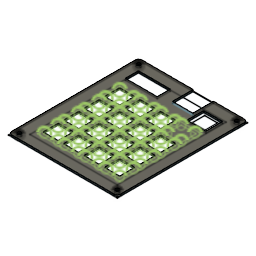
final (Autodesk Fusion 360 archive; units mm, degrees)
design "top"
part number: 2025-12-10-00-46-04-240
Autodesk Fusion 360 part; units mm, degrees
sketch "plate-2025-12-08T02_56_49.771Z" plane through (0, 0, 0) normal (0, 0, 1) x (1, 0, 0)
  line L0 (3.025, -2.525) -> (16.025, -2.525)
  line L1 (3.025, -16.525) -> (16.025, -16.525)
  line L2 (2.525, -3.025) -> (2.525, -16.025)
  line L3 (16.525, -3.025) -> (16.525, -16.025)
  arc A0 (3.025, -2.525) -> (2.525, -3.025) centre (3.025, -3.025) ccw
  arc A1 (16.525, -3.025) -> (16.025, -2.525) centre (16.025, -3.025) ccw
  arc A2 (2.525, -16.025) -> (3.025, -16.525) centre (3.025, -16.025) ccw
  arc A3 (16.025, -16.525) -> (16.525, -16.025) centre (16.025, -16.025) ccw
  line L4 (22.075, -2.525) -> (35.075, -2.525)
  line L5 (22.075, -16.525) -> (35.075, -16.525)
  line L6 (21.575, -3.025) -> (21.575, -16.025)
  line L7 (35.575, -3.025) -> (35.575, -16.025)
  arc A4 (22.075, -2.525) -> (21.575, -3.025) centre (22.075, -3.025) ccw
  arc A5 (35.575, -3.025) -> (35.075, -2.525) centre (35.075, -3.025) ccw
  arc A6 (21.575, -16.025) -> (22.075, -16.525) centre (22.075, -16.025) ccw
  arc A7 (35.075, -16.525) -> (35.575, -16.025) centre (35.075, -16.025) ccw
  line L8 (41.125, -2.525) -> (54.125, -2.525)
  line L9 (41.125, -16.525) -> (54.125, -16.525)
  line L10 (40.625, -3.025) -> (40.625, -16.025)
  line L11 (54.625, -3.025) -> (54.625, -16.025)
  arc A8 (41.125, -2.525) -> (40.625, -3.025) centre (41.125, -3.025) ccw
  arc A9 (54.625, -3.025) -> (54.125, -2.525) centre (54.125, -3.025) ccw
  arc A10 (40.625, -16.025) -> (41.125, -16.525) centre (41.125, -16.025) ccw
  arc A11 (54.125, -16.525) -> (54.625, -16.025) centre (54.125, -16.025) ccw
  line L12 (60.175, -2.525) -> (73.175, -2.525)
  line L13 (60.175, -16.525) -> (73.175, -16.525)
  line L14 (59.675, -3.025) -> (59.675, -16.025)
  line L15 (73.675, -3.025) -> (73.675, -16.025)
  arc A12 (60.175, -2.525) -> (59.675, -3.025) centre (60.175, -3.025) ccw
  arc A13 (73.675, -3.025) -> (73.175, -2.525) centre (73.175, -3.025) ccw
  arc A14 (59.675, -16.025) -> (60.175, -16.525) centre (60.175, -16.025) ccw
  arc A15 (73.175, -16.525) -> (73.675, -16.025) centre (73.175, -16.025) ccw
  line L16 (3.025, -21.575) -> (16.025, -21.575)
  line L17 (3.025, -35.575) -> (16.025, -35.575)
  line L18 (2.525, -22.075) -> (2.525, -35.075)
  line L19 (16.525, -22.075) -> (16.525, -35.075)
  arc A16 (3.025, -21.575) -> (2.525, -22.075) centre (3.025, -22.075) ccw
  arc A17 (16.525, -22.075) -> (16.025, -21.575) centre (16.025, -22.075) ccw
  arc A18 (2.525, -35.075) -> (3.025, -35.575) centre (3.025, -35.075) ccw
  arc A19 (16.025, -35.575) -> (16.525, -35.075) centre (16.025, -35.075) ccw
  line L20 (22.075, -21.575) -> (35.075, -21.575)
  line L21 (22.075, -35.575) -> (35.075, -35.575)
  line L22 (21.575, -22.075) -> (21.575, -35.075)
  line L23 (35.575, -22.075) -> (35.575, -35.075)
  arc A20 (22.075, -21.575) -> (21.575, -22.075) centre (22.075, -22.075) ccw
  arc A21 (35.575, -22.075) -> (35.075, -21.575) centre (35.075, -22.075) ccw
  arc A22 (21.575, -35.075) -> (22.075, -35.575) centre (22.075, -35.075) ccw
  arc A23 (35.075, -35.575) -> (35.575, -35.075) centre (35.075, -35.075) ccw
  line L24 (41.125, -21.575) -> (54.125, -21.575)
  line L25 (41.125, -35.575) -> (54.125, -35.575)
  line L26 (40.625, -22.075) -> (40.625, -35.075)
  line L27 (54.625, -22.075) -> (54.625, -35.075)
  arc A24 (41.125, -21.575) -> (40.625, -22.075) centre (41.125, -22.075) ccw
  arc A25 (54.625, -22.075) -> (54.125, -21.575) centre (54.125, -22.075) ccw
  arc A26 (40.625, -35.075) -> (41.125, -35.575) centre (41.125, -35.075) ccw
  arc A27 (54.125, -35.575) -> (54.625, -35.075) centre (54.125, -35.075) ccw
  line L28 (60.175, -21.575) -> (73.175, -21.575)
  line L29 (60.175, -35.575) -> (73.175, -35.575)
  line L30 (59.675, -22.075) -> (59.675, -35.075)
  line L31 (73.675, -22.075) -> (73.675, -35.075)
  arc A28 (60.175, -21.575) -> (59.675, -22.075) centre (60.175, -22.075) ccw
  arc A29 (73.675, -22.075) -> (73.175, -21.575) centre (73.175, -22.075) ccw
  arc A30 (59.675, -35.075) -> (60.175, -35.575) centre (60.175, -35.075) ccw
  arc A31 (73.175, -35.575) -> (73.675, -35.075) centre (73.175, -35.075) ccw
  line L32 (3.025, -40.625) -> (16.025, -40.625)
  line L33 (3.025, -54.625) -> (16.025, -54.625)
  line L34 (2.525, -41.125) -> (2.525, -54.125)
  line L35 (16.525, -41.125) -> (16.525, -54.125)
  arc A32 (3.025, -40.625) -> (2.525, -41.125) centre (3.025, -41.125) ccw
  arc A33 (16.525, -41.125) -> (16.025, -40.625) centre (16.025, -41.125) ccw
  arc A34 (2.525, -54.125) -> (3.025, -54.625) centre (3.025, -54.125) ccw
  arc A35 (16.025, -54.625) -> (16.525, -54.125) centre (16.025, -54.125) ccw
  line L36 (22.075, -40.625) -> (35.075, -40.625)
  line L37 (22.075, -54.625) -> (35.075, -54.625)
  line L38 (21.575, -41.125) -> (21.575, -54.125)
  line L39 (35.575, -41.125) -> (35.575, -54.125)
  arc A36 (22.075, -40.625) -> (21.575, -41.125) centre (22.075, -41.125) ccw
  arc A37 (35.575, -41.125) -> (35.075, -40.625) centre (35.075, -41.125) ccw
  arc A38 (21.575, -54.125) -> (22.075, -54.625) centre (22.075, -54.125) ccw
  arc A39 (35.075, -54.625) -> (35.575, -54.125) centre (35.075, -54.125) ccw
  line L40 (41.125, -40.625) -> (54.125, -40.625)
  line L41 (41.125, -54.625) -> (54.125, -54.625)
  line L42 (40.625, -41.125) -> (40.625, -54.125)
  line L43 (54.625, -41.125) -> (54.625, -54.125)
  arc A40 (41.125, -40.625) -> (40.625, -41.125) centre (41.125, -41.125) ccw
  arc A41 (54.625, -41.125) -> (54.125, -40.625) centre (54.125, -41.125) ccw
  arc A42 (40.625, -54.125) -> (41.125, -54.625) centre (41.125, -54.125) ccw
  arc A43 (54.125, -54.625) -> (54.625, -54.125) centre (54.125, -54.125) ccw
  line L44 (60.175, -40.625) -> (73.175, -40.625)
  line L45 (60.175, -54.625) -> (73.175, -54.625)
  line L46 (59.675, -41.125) -> (59.675, -54.125)
  line L47 (73.675, -41.125) -> (73.675, -54.125)
  arc A44 (60.175, -40.625) -> (59.675, -41.125) centre (60.175, -41.125) ccw
  arc A45 (73.675, -41.125) -> (73.175, -40.625) centre (73.175, -41.125) ccw
  arc A46 (59.675, -54.125) -> (60.175, -54.625) centre (60.175, -54.125) ccw
  arc A47 (73.175, -54.625) -> (73.675, -54.125) centre (73.175, -54.125) ccw
  line L48 (3.025, -59.675) -> (16.025, -59.675)
  line L49 (3.025, -73.675) -> (16.025, -73.675)
  line L50 (2.525, -60.175) -> (2.525, -73.175)
  line L51 (16.525, -60.175) -> (16.525, -73.175)
  arc A48 (3.025, -59.675) -> (2.525, -60.175) centre (3.025, -60.175) ccw
  arc A49 (16.525, -60.175) -> (16.025, -59.675) centre (16.025, -60.175) ccw
  arc A50 (2.525, -73.175) -> (3.025, -73.675) centre (3.025, -73.175) ccw
  arc A51 (16.025, -73.675) -> (16.525, -73.175) centre (16.025, -73.175) ccw
  line L52 (22.075, -59.675) -> (35.075, -59.675)
  line L53 (22.075, -73.675) -> (35.075, -73.675)
  line L54 (21.575, -60.175) -> (21.575, -73.175)
  line L55 (35.575, -60.175) -> (35.575, -73.175)
  arc A52 (22.075, -59.675) -> (21.575, -60.175) centre (22.075, -60.175) ccw
  arc A53 (35.575, -60.175) -> (35.075, -59.675) centre (35.075, -60.175) ccw
  arc A54 (21.575, -73.175) -> (22.075, -73.675) centre (22.075, -73.175) ccw
  arc A55 (35.075, -73.675) -> (35.575, -73.175) centre (35.075, -73.175) ccw
  line L56 (41.125, -59.675) -> (54.125, -59.675)
  line L57 (41.125, -73.675) -> (54.125, -73.675)
  line L58 (40.625, -60.175) -> (40.625, -73.175)
  line L59 (54.625, -60.175) -> (54.625, -73.175)
  arc A56 (41.125, -59.675) -> (40.625, -60.175) centre (41.125, -60.175) ccw
  arc A57 (54.625, -60.175) -> (54.125, -59.675) centre (54.125, -60.175) ccw
  arc A58 (40.625, -73.175) -> (41.125, -73.675) centre (41.125, -73.175) ccw
  arc A59 (54.125, -73.675) -> (54.625, -73.175) centre (54.125, -73.175) ccw
  line L60 (60.175, -59.675) -> (73.175, -59.675)
  line L61 (60.175, -73.675) -> (73.175, -73.675)
  line L62 (59.675, -60.175) -> (59.675, -73.175)
  line L63 (73.675, -60.175) -> (73.675, -73.175)
  arc A60 (60.175, -59.675) -> (59.675, -60.175) centre (60.175, -60.175) ccw
  arc A61 (73.675, -60.175) -> (73.175, -59.675) centre (73.175, -60.175) ccw
  arc A62 (59.675, -73.175) -> (60.175, -73.675) centre (60.175, -73.175) ccw
  arc A63 (73.175, -73.675) -> (73.675, -73.175) centre (73.175, -73.175) ccw
  line L64 (0, -76.2) -> (76.2, -76.2)
  line L65 (0, 0) -> (76.2, 0)
  line L66 (0, -76.2) -> (0, 0)
  line L67 (76.2, -76.2) -> (76.2, 0)
  line L68 (-2.995, 20.635) -> (78.195, 20.635)
  line L69 (78.195, 20.635) -> (78.195, -80.365)
  line L70 (78.195, -80.365) -> (-2.995, -80.365)
  line L71 (-2.995, -80.365) -> (-2.995, 20.635)
  line L72 (62.965, 16.055) -> (74.965, 16.055)
  line L73 (74.965, 16.055) -> (74.965, 4.455)
  line L74 (74.965, 4.455) -> (62.965, 4.455)
  line L75 (62.965, 4.455) -> (62.965, 16.055)
  line L76 (60.065, 18.055) -> (77.565, 18.055)
  line L77 (77.565, 18.055) -> (77.565, 2.655)
  line L78 (77.565, 2.655) -> (60.065, 2.655)
  line L79 (60.065, 2.655) -> (60.065, 18.055)
  line L80 (-2.28, 19.7) -> (27.22, 19.7)
  line L81 (27.22, 19.7) -> (27.22, 7.7)
  line L82 (27.22, 7.7) -> (-2.28, 7.7)
  line L83 (-2.28, 7.7) -> (-2.28, 19.7)
  line L84 (-12.495, 30.135) -> (88.695, 30.135)
  line L85 (88.695, 30.135) -> (88.695, -90.865)
  line L86 (88.695, -90.865) -> (-12.495, -90.865)
  line L87 (-12.495, -90.865) -> (-12.495, 30.135)
  circle A64 centre (-7.495, 25.135) radius 1.7
  circle A65 centre (-7.495, -85.865) radius 1.7
  circle A66 centre (83.695, -85.865) radius 1.7
  circle A67 centre (83.695, 25.135) radius 1.7
  line L88 (38.235, 30.135) -> (57.064, 30.135)
  line L89 (57.064, 30.135) -> (57.064, 11)
  line L90 (57.064, 11) -> (38.235, 11)
  line L91 (38.235, 11) -> (38.235, 30.135)
  dimension "d3" = 101
  dimension "d4" = 81.19
  dimension "d6" = 1.995
  dimension "d7" = 4.165
  dimension "d11" = 12
  dimension "d12" = 11.6
  dimension "d16" = 15.4
  dimension "d17" = 17.5
  dimension "d18" = 2.9
  dimension "d19" = 1.8
  dimension "d22" = 29.5
  dimension "d23" = 12
  dimension "d25" = 0.935
  dimension "d29" = 0.715
  dimension "d33" = 9.5
  dimension "d34" = 3.4
  dimension "d35" = 5
  dimension "d36" = 5
  dimension "d37" = 3.4
  dimension "d38" = 5
  dimension "d39" = 5
  dimension "d40" = 3.4
  dimension "d41" = 5
  dimension "d42" = 5
  dimension "d43" = 3.4
  dimension "d44" = 5
  dimension "d45" = 5
  dimension "d46" = 41.23
  dimension "d48" = 21.131
  dimension "d49" = 18.829
  dimension "d53" = 2.58
  dimension "d55" = 0.63
  dimension "d65" = 121
  dimension "d66" = 9.5
  dimension "d67" = 10.5
  constraint horizontal L68
  constraint vertical L69
  constraint horizontal L70
  constraint vertical L71
  constraint horizontal L72
  constraint vertical L73
  constraint horizontal L74
  constraint vertical L75
  constraint horizontal L76
  constraint vertical L77
  constraint horizontal L78
  constraint vertical L79
  constraint horizontal L80
  constraint vertical L81
  constraint horizontal L82
  constraint vertical L83
  constraint horizontal L84
  constraint vertical L85
  constraint horizontal L86
  constraint vertical L87
  constraint horizontal L88
  constraint vertical L89
  constraint horizontal L90
  constraint vertical L91
  constraint coincident L84 L88.start
  measures "d3" distance of L68.end L69.end
  measures "d4" distance of L69.end L70.end
  measures "d6" distance of L67 L69
  measures "d7" distance of L64 L70
  measures "d11" distance of L72.start L72.end
  measures "d12" distance of L72.start L74.end
  measures "d16" distance of L76.start L78.end
  measures "d17" distance of L77.end L78.end
  measures "d18" distance of L75 L79
  measures "d19" distance of L74 L78
  measures "d22" distance of L81.end L82.end
  measures "d23" distance of L80.end L81.end
  measures "d25" distance of L68 L80
  measures "d29" distance of L71 L83
  measures "d33" distance of L68 L84
  measures "d34" diameter of A64
  measures "d35" distance of L84 A64.centre
  measures "d36" distance of L87 A64.centre
  measures "d37" diameter of A65
  measures "d38" distance of L86 A65.centre
  measures "d39" distance of L87 A65.centre
  measures "d40" diameter of A66
  measures "d41" distance of L86 A66.centre
  measures "d42" distance of L85 A66.centre
  measures "d43" diameter of A67
  measures "d44" distance of L84 A67.centre
  measures "d45" distance of L85 A67.centre
  measures "d46" distance of L71 L90.end
  measures "d48" distance of L69 L89.end
  measures "d49" distance of L89.end L90.end
  measures "d53" vertical distance of L68.end L76.end
  measures "d55" distance of L69 L77
  measures "d65" distance of L84.end L85.end
  measures "d66" distance of L71 L87
  measures "d67" distance of L69 L85
extrude "Extrude1" add sketch "plate-2025-12-08T02_56_49.771Z" along normal blind 1.5 contours L68 L69 L70 L71 L89 L90 L91
extrude "Extrude2" add sketch "plate-2025-12-08T02_56_49.771Z" along normal blind 1.5 contours L68 L69 L70 L71 L84 L85 L86 L87 L89 L91
extrude "Extrude3" add sketch "plate-2025-12-08T02_56_49.771Z" along normal blind 1.5 contours L64 L65 L66 L67
fillet "Fillet1" radius 3 4 edges at (88.695, -90.865, 0.75) (88.695, 30.135, 0.75) (-12.495, 30.135, 0.75) (-12.495, -90.865, 0.75)
sketch "Sketch2" plane through (0, 0, 1.5) normal (0, 0, 1) x (1, 0, 0)
sketch "Sketch3" plane through (0, 0, 1.5) normal (0, 0, 1) x (-1, 0, 0)
  arc A0 (12.495, 87.865) -> (9.495, 90.865) centre (9.495, 87.865) ccw
  line L0 (9.495, 90.865) -> (-85.695, 90.865)
  arc A1 (-85.695, 90.865) -> (-88.695, 87.865) centre (-85.695, 87.865) ccw
  line L1 (-88.695, 87.865) -> (-88.695, -27.135)
  arc A2 (-88.695, -27.135) -> (-85.695, -30.135) centre (-85.695, -27.135) ccw
  line L2 (-85.695, -30.135) -> (-57.064, -30.135)
  line L3 (-57.064, -30.135) -> (-57.064, -11)
  line L4 (-57.064, -11) -> (-38.235, -11)
  line L5 (-38.235, -11) -> (-38.235, -30.135)
  line L6 (-38.235, -30.135) -> (9.495, -30.135)
  arc A3 (9.495, -30.135) -> (12.495, -27.135) centre (9.495, -27.135) ccw
  line L7 (12.495, -27.135) -> (12.495, 87.865)
  arc A4 (-41.125, 2.525) -> (-40.625, 3.025) centre (-41.125, 3.025) ccw
  line L8 (-41.125, 2.525) -> (-54.125, 2.525)
  arc A5 (-54.625, 3.025) -> (-54.125, 2.525) centre (-54.125, 3.025) ccw
  line L9 (-54.625, 3.025) -> (-54.625, 16.025)
  arc A6 (-54.125, 16.525) -> (-54.625, 16.025) centre (-54.125, 16.025) ccw
  line L10 (-54.125, 16.525) -> (-41.125, 16.525)
  arc A7 (-40.625, 16.025) -> (-41.125, 16.525) centre (-41.125, 16.025) ccw
  line L11 (-40.625, 16.025) -> (-40.625, 3.025)
  arc A8 (-3.025, 59.675) -> (-2.525, 60.175) centre (-3.025, 60.175) ccw
  line L12 (-3.025, 59.675) -> (-16.025, 59.675)
  arc A9 (-16.525, 60.175) -> (-16.025, 59.675) centre (-16.025, 60.175) ccw
  line L13 (-16.525, 60.175) -> (-16.525, 73.175)
  arc A10 (-16.025, 73.675) -> (-16.525, 73.175) centre (-16.025, 73.175) ccw
  line L14 (-16.025, 73.675) -> (-3.025, 73.675)
  arc A11 (-2.525, 73.175) -> (-3.025, 73.675) centre (-3.025, 73.175) ccw
  line L15 (-2.525, 73.175) -> (-2.525, 60.175)
  arc A12 (-60.175, 2.525) -> (-59.675, 3.025) centre (-60.175, 3.025) ccw
  line L16 (-60.175, 2.525) -> (-73.175, 2.525)
  arc A13 (-73.675, 3.025) -> (-73.175, 2.525) centre (-73.175, 3.025) ccw
  line L17 (-73.675, 3.025) -> (-73.675, 16.025)
  arc A14 (-73.175, 16.525) -> (-73.675, 16.025) centre (-73.175, 16.025) ccw
  line L18 (-73.175, 16.525) -> (-60.175, 16.525)
  arc A15 (-59.675, 16.025) -> (-60.175, 16.525) centre (-60.175, 16.025) ccw
  line L19 (-59.675, 16.025) -> (-59.675, 3.025)
  arc A16 (-22.075, 21.575) -> (-21.575, 22.075) centre (-22.075, 22.075) ccw
  line L20 (-22.075, 21.575) -> (-35.075, 21.575)
  arc A17 (-35.575, 22.075) -> (-35.075, 21.575) centre (-35.075, 22.075) ccw
  line L21 (-35.575, 22.075) -> (-35.575, 35.075)
  arc A18 (-35.075, 35.575) -> (-35.575, 35.075) centre (-35.075, 35.075) ccw
  line L22 (-35.075, 35.575) -> (-22.075, 35.575)
  arc A19 (-21.575, 35.075) -> (-22.075, 35.575) centre (-22.075, 35.075) ccw
  line L23 (-21.575, 35.075) -> (-21.575, 22.075)
  arc A20 (-41.125, 40.625) -> (-40.625, 41.125) centre (-41.125, 41.125) ccw
  line L24 (-41.125, 40.625) -> (-54.125, 40.625)
  arc A21 (-54.625, 41.125) -> (-54.125, 40.625) centre (-54.125, 41.125) ccw
  line L25 (-54.625, 41.125) -> (-54.625, 54.125)
  arc A22 (-54.125, 54.625) -> (-54.625, 54.125) centre (-54.125, 54.125) ccw
  line L26 (-54.125, 54.625) -> (-41.125, 54.625)
  arc A23 (-40.625, 54.125) -> (-41.125, 54.625) centre (-41.125, 54.125) ccw
  line L27 (-40.625, 54.125) -> (-40.625, 41.125)
  arc A24 (-22.075, 40.625) -> (-21.575, 41.125) centre (-22.075, 41.125) ccw
  line L28 (-22.075, 40.625) -> (-35.075, 40.625)
  arc A25 (-35.575, 41.125) -> (-35.075, 40.625) centre (-35.075, 41.125) ccw
  line L29 (-35.575, 41.125) -> (-35.575, 54.125)
  arc A26 (-35.075, 54.625) -> (-35.575, 54.125) centre (-35.075, 54.125) ccw
  line L30 (-35.075, 54.625) -> (-22.075, 54.625)
  arc A27 (-21.575, 54.125) -> (-22.075, 54.625) centre (-22.075, 54.125) ccw
  line L31 (-21.575, 54.125) -> (-21.575, 41.125)
  arc A28 (-41.125, 59.675) -> (-40.625, 60.175) centre (-41.125, 60.175) ccw
  line L32 (-41.125, 59.675) -> (-54.125, 59.675)
  arc A29 (-54.625, 60.175) -> (-54.125, 59.675) centre (-54.125, 60.175) ccw
  line L33 (-54.625, 60.175) -> (-54.625, 73.175)
  arc A30 (-54.125, 73.675) -> (-54.625, 73.175) centre (-54.125, 73.175) ccw
  line L34 (-54.125, 73.675) -> (-41.125, 73.675)
  arc A31 (-40.625, 73.175) -> (-41.125, 73.675) centre (-41.125, 73.175) ccw
  line L35 (-40.625, 73.175) -> (-40.625, 60.175)
  arc A32 (-3.025, 2.525) -> (-2.525, 3.025) centre (-3.025, 3.025) ccw
  line L36 (-3.025, 2.525) -> (-16.025, 2.525)
  arc A33 (-16.525, 3.025) -> (-16.025, 2.525) centre (-16.025, 3.025) ccw
  line L37 (-16.525, 3.025) -> (-16.525, 16.025)
  arc A34 (-16.025, 16.525) -> (-16.525, 16.025) centre (-16.025, 16.025) ccw
  line L38 (-16.025, 16.525) -> (-3.025, 16.525)
  arc A35 (-2.525, 16.025) -> (-3.025, 16.525) centre (-3.025, 16.025) ccw
  line L39 (-2.525, 16.025) -> (-2.525, 3.025)
  arc A36 (-60.175, 21.575) -> (-59.675, 22.075) centre (-60.175, 22.075) ccw
  line L40 (-60.175, 21.575) -> (-73.175, 21.575)
  arc A37 (-73.675, 22.075) -> (-73.175, 21.575) centre (-73.175, 22.075) ccw
  line L41 (-73.675, 22.075) -> (-73.675, 35.075)
  arc A38 (-73.175, 35.575) -> (-73.675, 35.075) centre (-73.175, 35.075) ccw
  line L42 (-73.175, 35.575) -> (-60.175, 35.575)
  arc A39 (-59.675, 35.075) -> (-60.175, 35.575) centre (-60.175, 35.075) ccw
  line L43 (-59.675, 35.075) -> (-59.675, 22.075)
  arc A40 (-60.175, 59.675) -> (-59.675, 60.175) centre (-60.175, 60.175) ccw
  line L44 (-60.175, 59.675) -> (-73.175, 59.675)
  arc A41 (-73.675, 60.175) -> (-73.175, 59.675) centre (-73.175, 60.175) ccw
  line L45 (-73.675, 60.175) -> (-73.675, 73.175)
  arc A42 (-73.175, 73.675) -> (-73.675, 73.175) centre (-73.175, 73.175) ccw
  line L46 (-73.175, 73.675) -> (-60.175, 73.675)
  arc A43 (-59.675, 73.175) -> (-60.175, 73.675) centre (-60.175, 73.175) ccw
  line L47 (-59.675, 73.175) -> (-59.675, 60.175)
  arc A44 (-60.175, 40.625) -> (-59.675, 41.125) centre (-60.175, 41.125) ccw
  line L48 (-60.175, 40.625) -> (-73.175, 40.625)
  arc A45 (-73.675, 41.125) -> (-73.175, 40.625) centre (-73.175, 41.125) ccw
  line L49 (-73.675, 41.125) -> (-73.675, 54.125)
  arc A46 (-73.175, 54.625) -> (-73.675, 54.125) centre (-73.175, 54.125) ccw
  line L50 (-73.175, 54.625) -> (-60.175, 54.625)
  arc A47 (-59.675, 54.125) -> (-60.175, 54.625) centre (-60.175, 54.125) ccw
  line L51 (-59.675, 54.125) -> (-59.675, 41.125)
  arc A48 (-41.125, 21.575) -> (-40.625, 22.075) centre (-41.125, 22.075) ccw
  line L52 (-41.125, 21.575) -> (-54.125, 21.575)
  arc A49 (-54.625, 22.075) -> (-54.125, 21.575) centre (-54.125, 22.075) ccw
  line L53 (-54.625, 22.075) -> (-54.625, 35.075)
  arc A50 (-54.125, 35.575) -> (-54.625, 35.075) centre (-54.125, 35.075) ccw
  line L54 (-54.125, 35.575) -> (-41.125, 35.575)
  arc A51 (-40.625, 35.075) -> (-41.125, 35.575) centre (-41.125, 35.075) ccw
  line L55 (-40.625, 35.075) -> (-40.625, 22.075)
  arc A52 (-22.075, 2.525) -> (-21.575, 3.025) centre (-22.075, 3.025) ccw
  line L56 (-22.075, 2.525) -> (-35.075, 2.525)
  arc A53 (-35.575, 3.025) -> (-35.075, 2.525) centre (-35.075, 3.025) ccw
  line L57 (-35.575, 3.025) -> (-35.575, 16.025)
  arc A54 (-35.075, 16.525) -> (-35.575, 16.025) centre (-35.075, 16.025) ccw
  line L58 (-35.075, 16.525) -> (-22.075, 16.525)
  arc A55 (-21.575, 16.025) -> (-22.075, 16.525) centre (-22.075, 16.025) ccw
  line L59 (-21.575, 16.025) -> (-21.575, 3.025)
  arc A56 (-3.025, 40.625) -> (-2.525, 41.125) centre (-3.025, 41.125) ccw
  line L60 (-3.025, 40.625) -> (-16.025, 40.625)
  arc A57 (-16.525, 41.125) -> (-16.025, 40.625) centre (-16.025, 41.125) ccw
  line L61 (-16.525, 41.125) -> (-16.525, 54.125)
  arc A58 (-16.025, 54.625) -> (-16.525, 54.125) centre (-16.025, 54.125) ccw
  line L62 (-16.025, 54.625) -> (-3.025, 54.625)
  arc A59 (-2.525, 54.125) -> (-3.025, 54.625) centre (-3.025, 54.125) ccw
  line L63 (-2.525, 54.125) -> (-2.525, 41.125)
  arc A60 (-3.025, 21.575) -> (-2.525, 22.075) centre (-3.025, 22.075) ccw
  line L64 (-3.025, 21.575) -> (-16.025, 21.575)
  arc A61 (-16.525, 22.075) -> (-16.025, 21.575) centre (-16.025, 22.075) ccw
  line L65 (-16.525, 22.075) -> (-16.525, 35.075)
  arc A62 (-16.025, 35.575) -> (-16.525, 35.075) centre (-16.025, 35.075) ccw
  line L66 (-16.025, 35.575) -> (-3.025, 35.575)
  arc A63 (-2.525, 35.075) -> (-3.025, 35.575) centre (-3.025, 35.075) ccw
  line L67 (-2.525, 35.075) -> (-2.525, 22.075)
  arc A64 (-22.075, 59.675) -> (-21.575, 60.175) centre (-22.075, 60.175) ccw
  line L68 (-22.075, 59.675) -> (-35.075, 59.675)
  arc A65 (-35.575, 60.175) -> (-35.075, 59.675) centre (-35.075, 60.175) ccw
  line L69 (-35.575, 60.175) -> (-35.575, 73.175)
  arc A66 (-35.075, 73.675) -> (-35.575, 73.175) centre (-35.075, 73.175) ccw
  line L70 (-35.075, 73.675) -> (-22.075, 73.675)
  arc A67 (-21.575, 73.175) -> (-22.075, 73.675) centre (-22.075, 73.175) ccw
  line L71 (-21.575, 73.175) -> (-21.575, 60.175)
  circle A68 centre (7.495, -25.135) radius 1.7
  circle A69 centre (7.495, 85.865) radius 1.7
  circle A70 centre (-83.695, -25.135) radius 1.7
  circle A71 centre (-83.695, 85.865) radius 1.7
  line L72 (-27.22, -7.7) -> (2.28, -7.7)
  line L73 (2.28, -7.7) -> (2.28, -19.7)
  line L74 (2.28, -19.7) -> (-27.22, -19.7)
  line L75 (-27.22, -19.7) -> (-27.22, -7.7)
  line L76 (-77.565, -2.655) -> (-60.065, -2.655)
  line L77 (-60.065, -2.655) -> (-60.065, -18.055)
  line L78 (-60.065, -18.055) -> (-77.565, -18.055)
  line L79 (-77.565, -18.055) -> (-77.565, -2.655)
extrude "Extrude4" add sketch "Sketch3" along normal blind 1.5 from surface at -1.5 contours A12 L16 A13 L17 A14 L18 A15 L19
sketch "Sketch4" plane through (0, 0, 0) normal (0, 0, 1) x (1, 0, 0)
